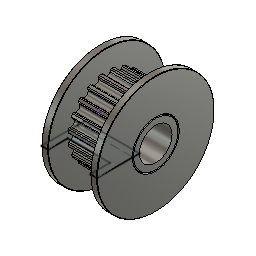
Idler plate R1 v7 (Autodesk Fusion 360 archive; units mm, degrees)
design "GT2 20T 6mm belt Ider"
Autodesk Fusion 360 part; units mm, degrees
sketch "Sketch5" plane through (0, 0, 0) normal (0, 1, 0) x (1, 0, 0) in component "GT2_20T_5mmBore_10mmBelt Idler v3 v1"
  line L0 (0, -9) -> (1, -9)
  line L1 (1, -9) -> (1, -6)
  line L2 (1, -6) -> (7.5, -6)
  line L3 (7.5, -6) -> (7.5, -9)
  line L4 (7.5, -9) -> (8.5, -9)
  line L5 (8.5, -9) -> (8.5, -3.6)
  line L6 (8.5, -3.6) -> (8.4, -3.5)
  line L7 (8.4, -3.5) -> (8.5, -3.4)
  line L8 (8.5, -3.4) -> (8.5, -2.5)
  line L9 (8.5, -2.5) -> (0, -2.5)
  line L10 (8.4, -3.5) -> (0.1, -3.5) construction
  line L11 (0, -3.4) -> (0.1, -3.5)
  line L12 (0.1, -3.5) -> (0, -3.6)
  line L13 (0, -2.5) -> (0, -3.4)
  line L14 (0, -3.6) -> (0, -9)
  dimension "d24" = 90
  dimension "d25" = 3.5
  dimension "d26" = 2.5
  dimension "d30" = 1
  dimension "d31" = 6.5
  dimension "d32" = 0.1
  dimension "d33" = 1
  dimension "d35" = 9
  dimension "d36" = 9
  dimension "d48" = 8.5
  dimension "d49" = 0.1
  dimension "d1" = 1
  constraint vertical L13
  constraint horizontal L0
  constraint horizontal L2
  constraint vertical L1
  constraint vertical L3
  constraint horizontal L9
  constraint vertical L8
  constraint vertical L5
  constraint horizontal L4
  constraint coincident origin L13
  constraint collinear L5 L8
  constraint horizontal L10
  constraint symmetric L6 L7 L10
  constraint coincident L12.end L13
  constraint perpendicular L11 L12
  constraint coincident L10.end L11.end
  constraint collinear L13 L14
  constraint symmetric L10 L11 L12
  measures "d24" angle of L6 L7
  measures "d25" distance of L2 L9
  measures "d26" distance of origin L9
  measures "d30" distance of L6.end L9
  measures "d31" horizontal distance of L1.end L2.end
  measures "d32" distance of L6.end L8
  measures "d33" horizontal distance of L0.start L0.end
  measures "d35" distance of origin L0
  measures "d36" distance of origin L4
  measures "d48" horizontal distance of L8.end L9.end
  measures "d49" distance of L10.end L13
  measures "d1" distance of L3.end L4.end
revolve "Revolve1" add sketch "Sketch5" angle 360 about axis through (1.75, 0, 0) along (1, 0, 0) in component "GT2_20T_5mmBore_10mmBelt Idler v3 v1"
sketch "Sketch4" plane through (7.5, 0, 0) normal (-1, 0, 0) x (0, 0, 1) in component "GT2_20T_5mmBore_10mmBelt Idler v3 v1"
  line L0 (0, 0) -> (0, 6) construction
  circle A0 centre (0, 0) radius 5.25 construction
  circle A1 centre (0, 0) radius 5.805 construction
  arc A2 (-0.4989, 5.5618) -> (0, 5.25) centre (0, 5.805) ccw
  arc A3 (-0.5996, 5.97) -> (-0.4989, 5.5618) centre (0.4, 6) ccw
  arc A4 (0.4989, 5.5618) -> (0.5995, 5.97) centre (-0.4, 6) ccw
  arc A5 (0, 5.25) -> (0.4989, 5.5618) centre (0, 5.805) ccw
  circle A6 centre (0, 0) radius 9
  circle A7 centre (0, 0) radius 6
  dimension "d14" = 0.4
  dimension "d16" = 1
  dimension "d18" = 0.555
  dimension "d50" = 0.75
  constraint vertical L0
  constraint coincident A2.centre L0
  constraint tangent A0 A2
  constraint coincident A2.centre A1
  constraint tangent A2 A3
  constraint coincident L0 A2.end
  constraint symmetric L0 A2 A5
  constraint symmetric L0 A3 A4
  constraint symmetric L0 A2.end A5.start
  constraint symmetric L0 A2.start A4.start
  constraint symmetric L0 A3.start A4.end
  constraint coincident L0.end A7
  constraint coincident L0.start A0.centre
  constraint coincident A3.start A7
  measures "d14" distance of L0 A3.centre
  measures "d16" radius of A3
  measures "d18" radius of A2
  measures "d50" distance of L0.end A2.end
extrude "Extrude5" cut sketch "Sketch4" along normal up to surface (6.5 mm away) contours A2 A3 A4 A5 A7 picked at (0, 5.7478) in component "GT2_20T_5mmBore_10mmBelt Idler v3 v1"
fillet "Fillet1" radius 0.15 2 edges at (4.25, 5.97, -0.5996) (4.25, 5.97, 0.5995) in component "GT2_20T_5mmBore_10mmBelt Idler v3 v1"
pattern_circular "C-Pattern1" count 20 over 360 about axis through (1.75, 0, 0) along (1, 0, 0) of "Extrude5", "Fillet1" in component "GT2_20T_5mmBore_10mmBelt Idler v3 v1"
chamfer "Chamfer2" distance 0.06 angle 45 4 edges at (0, -3.2545, -8.3909) (1, -3.2545, -8.3909) (7.5, -3.2545, -8.3909) (8.5, -3.2545, -8.3909) in component "GT2_20T_5mmBore_10mmBelt Idler v3 v1"
component "GT2_20T_5mmBore_10mmBelt Idler v3 v1" placed x (1, 0, 0) y (0, 1, 0) z (0, 0, 1) at (0, 0, 0)
equation "d36 = d35"
named bodies: "GT2-16T-3Bore"
